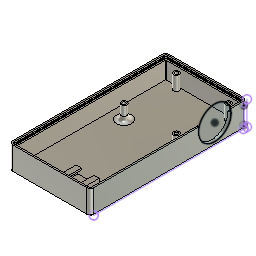
Boitier rover RTK (Autodesk Fusion 360 design; units mm, degrees)
Autodesk Fusion 360 part; units mm, degrees
sketch "Esquisse1" plane through (0, 0, 0) normal (0, 0, 1) x (1, 0, 0) in component "Face Antenne"
  line L0 (32, -67.5) -> (-32, -67.5)
  line L1 (-35, -64.5) -> (-35, 64.5)
  line L2 (-32, 67.5) -> (32, 67.5)
  line L3 (35, 64.5) -> (35, -64.5)
  line L4 (35, -67.5) -> (-35, 67.5) construction
  line L5 (-35, -67.5) -> (35, 67.5) construction
  arc A0 (-32, 67.5) -> (-35, 64.5) centre (-32, 64.5) ccw
  arc A1 (-35, -64.5) -> (-32, -67.5) centre (-32, -64.5) ccw
  arc A2 (32, -67.5) -> (35, -64.5) centre (32, -64.5) ccw
  arc A3 (35, 64.5) -> (32, 67.5) centre (32, 64.5) ccw
  dimension "d31" = 70
  dimension "d32" = 135
  dimension "d33" = 3
  constraint horizontal L0
  constraint perpendicular L0 L1
  constraint parallel L0 L2
  constraint parallel L1 L3
  constraint coincident L4 origin
  constraint coincident L5 origin
  constraint coincident L4.end L2
  constraint coincident L4.end L1
  constraint tangent L2 A0
  constraint tangent L1 A0
  constraint coincident L5.start L1
  constraint coincident L5.start L0
  constraint tangent L1 A1
  constraint tangent L0 A1
  constraint equal A0 A1
  constraint coincident L4.start L3
  constraint coincident L4.start L0
  constraint tangent L3 A2
  constraint tangent L0 A2
  constraint equal A0 A2
  constraint coincident L5.end L3
  constraint coincident L5.end L2
  constraint tangent L3 A3
  constraint tangent L2 A3
  constraint equal A0 A3
  measures "d31" distance of L4.end L5.end
  measures "d32" distance of L5.start L4.end
  measures "d33" radius of A0
extrude "Extrusion1" add sketch "Esquisse1" along normal blind 2.7 makes body 1 in component "Face Antenne"
sketch "Esquisse2" plane through (0, 0, 0) normal (0, 1, 0) x (1, 0, 0) in component "Face Antenne"
  line L0 (35, 0) -> (35, -20.7)
  line L1 (35, -20.7) -> (33.6, -20.7)
  line L2 (33.6, -20.7) -> (33.6, -19.2)
  line L3 (33.6, -19.2) -> (33.8, -19.2)
  line L4 (33.8, -19.2) -> (33.8, -18.2)
  line L5 (33.8, -18.2) -> (33.6, -18.2)
  line L6 (33.6, -18.2) -> (33.6, -17.7)
  line L7 (33.6, -17.7) -> (32.3, -17.7)
  line L8 (32.3, -17.7) -> (32.3, 0)
  line L9 (32.3, 0) -> (35, 0)
  line L10 (35, 0) -> (35, -2.7)
  line L11 (32, 0) -> (-32, 0)
  dimension "d36" = 2.7
  dimension "d37" = 1.4
  dimension "d38" = 1
  dimension "d39" = 0.5
  dimension "d41" = 0.2
  dimension "d42" = 20.7
  dimension "d131" = 1.5
  constraint vertical L0
  constraint perpendicular L0 L1
  constraint perpendicular L1 L2
  constraint perpendicular L2 L3
  constraint perpendicular L3 L4
  constraint perpendicular L4 L5
  constraint perpendicular L5 L6
  constraint perpendicular L6 L7
  constraint perpendicular L7 L8
  constraint perpendicular L0 L9
  constraint collinear L0 L10
  constraint collinear L9 L11
  constraint collinear L2 L6
  measures "d36" distance of L0.start L8.end
  measures "d37" distance of L0.end L1.end
  measures "d38" distance of L3.end L4.end
  measures "d39" distance of L5.end L6.end
  measures "d41" distance of L2.end L3.end
  measures "d42" distance of L0.start L0.end
  measures "d131" distance of L1.end L2.end
sweep "Balayage1" add profiles "Esquisse2" path "Esquisse1" along A2 L0 A1 L1 A0 L2 A3 L3 section 1 bodies 1 in component "Face Antenne"
sketch "Esquisse1 (2)" plane through (0, 0, 0) normal (0, 0, 1) x (1, 0, 0) in component "Face batterie"
  line L0 (-35, -64.5) -> (-35, 64.5)
  line L1 (35, 64.5) -> (35, -64.5)
  line L2 (-32, 67.5) -> (32, 67.5)
  arc A0 (-32, 67.5) -> (-35, 64.5) centre (-32, 64.5) ccw
  arc A1 (35, 64.5) -> (32, 67.5) centre (32, 64.5) ccw
  arc A2 (32, -67.5) -> (35, -64.5) centre (32, -64.5) ccw
  line L3 (32, -67.5) -> (-32, -67.5)
  arc A3 (-35, -64.5) -> (-32, -67.5) centre (-32, -64.5) ccw
  point P0 (-32, 64.5)
extrude "Extrusion1'" add sketch "Esquisse1 (2)" against normal blind 2.7 separate body makes body 2 in component "Face batterie"
sketch "Esquisse2 (2)" plane through (0, 0, 0) normal (0, 1, 0) x (1, 0, 0) in component "Face batterie"
  line L0 (35, 0) -> (35, 19.29)
  line L1 (35, 19.29) -> (33.4, 19.29)
  line L2 (33.4, 22.29) -> (32.3, 22.29)
  line L3 (32.3, 22.29) -> (32.3, 0)
  line L4 (32.3, 0) -> (35, 0)
  line L5 (33.8, 20.8) -> (33.8, 21.8)
  line L6 (32.3, 40) -> (35, 40)
  line L7 (32.3, 22.3) -> (32.3, 40)
  line L8 (32, 0) -> (-32, 0)
  line L9 (33.4, 21.7) -> (33.5, 21.7)
  line L10 (33.7, 21.5) -> (33.7, 21.1)
  line L11 (33.5, 20.9) -> (33.4, 20.9)
  line L12 (33.4, 19.29) -> (33.4, 20.9)
  line L13 (33.4, 21.7) -> (33.4, 22.29)
  line L14 (33.6, 19.3) -> (33.6, 20.8)
  line L15 (35, 19.3) -> (33.6, 19.3)
  line L16 (33.6, 22.3) -> (32.3, 22.3)
  line L17 (33.6, 20.8) -> (33.8, 20.8)
  line L18 (33.8, 21.8) -> (33.6, 21.8)
  arc A0 (33.7, 21.5) -> (33.5, 21.7) centre (33.5, 21.5) ccw
  arc A1 (33.5, 20.9) -> (33.7, 21.1) centre (33.5, 21.1) ccw
  dimension "d151" = 0.01
  dimension "d152" = 0.01
  dimension "d153" = 0.1
  dimension "d154" = 0.1
  dimension "d155" = 0.2
  dimension "d156" = 0.1
  dimension "d157" = 0.2
  constraint vertical L0
  constraint perpendicular L0 L1
  constraint perpendicular L1 L12
  constraint perpendicular L2 L3
  constraint perpendicular L0 L4
  constraint equal L4 L6
  constraint collinear L3 L7
  constraint collinear L4 L8
  constraint coincident L9.start L12
  constraint perpendicular L9 L12
  constraint perpendicular L9 L10
  constraint perpendicular L11 L12
  constraint vertical L13
  constraint coincident L2.end L7
  constraint tangent L9 A0
  constraint tangent L10 A0
  constraint tangent L11 A1
  constraint tangent L10 A1
  constraint equal A0 A1
  measures "d151" distance of L1 L15
  measures "d152" distance of L2 L16
  measures "d153" distance of L11 L17
  measures "d154" distance of L9 L18
  measures "d155" distance of L12 L14
  measures "d156" distance of L5 L10
  measures "d157" radius of A0
sweep "Balayage1'" add profiles "Esquisse2 (2)" path "Esquisse1 (2)" along L1 A1 L2 A0 L0 A3 L3 A2 section 1 bodies 2 in component "Face batterie"
sketch "Esquisse5" plane through (35, 0, 0) normal (1, 0, 0) x (0, 1, 0)
  line L0 (-64.5, 0) -> (64.5, 0)
  line L1 (64.5, 0) -> (64.5, 20.7)
  line L2 (64.5, 20.7) -> (-64.5, 20.7)
  line L3 (-64.5, 20.7) -> (-64.5, 0)
  line L4 (67.5, 0) -> (67.5, 20.7)
  line L5 (64.5, 0) -> (-64.5, 0)
  circle A0 centre (39.8, 17) radius 14
  line L6 (64.8, 2.7) -> (64.8, 17.7)
  line L7 (64.8, 17.7) -> (64.8, 2.7)
  dimension "d222" = 28
  dimension "d223" = 25
  dimension "d224" = 17
  measures "d222" diameter of A0
  measures "d223" distance of A0.centre L6
  measures "d224" distance of L5 A0.centre
extrude "Extrusion7" cut sketch "Esquisse5" against normal up to surface (2.7 mm away) contours L2 A0 | L2 A0 bodies 1 in component "Face Antenne"
extrude "Extrusion4" add sketch "Esquisse1" along normal blind 3 bodies 1 in component "Face Antenne"
sketch "Esquisse6" plane through (0, 0, 3) normal (0, 0, 1) x (-1, 0, 0) in component "Face Antenne"
  arc A0 (-32.3, -64.5) -> (-32, -64.8) centre (-32, -64.5) ccw
  line L0 (-32, -64.8) -> (32, -64.8)
  arc A1 (32, -64.8) -> (32.3, -64.5) centre (32, -64.5) ccw
  line L1 (32.3, -64.5) -> (32.3, 64.5)
  arc A2 (32.3, 64.5) -> (32, 64.8) centre (32, 64.5) ccw
  line L2 (32, 64.8) -> (-32, 64.8)
  arc A3 (-32, 64.8) -> (-32.3, 64.5) centre (-32, 64.5) ccw
  line L3 (-32.3, 64.5) -> (-32.3, -39.8)
  line L4 (-32.3, -39.8) -> (-32.3, -64.5)
  circle A4 centre (20.7, -62.3) radius 2.5
  circle A5 centre (-24.3, -62.3) radius 2.5
  circle A6 centre (20.7, -17.3) radius 2.5
  circle A7 centre (-24.3, -17.3) radius 2.5
  dimension "d87" = 45
  dimension "d88" = 45
  dimension "d90" = 8
  dimension "d211" = 2.5
  constraint equal A4 A5
  constraint equal A4 A6
  constraint equal A6 A7
  constraint vertical A5.centre A7.centre
  constraint vertical A4.centre A6.centre
  constraint horizontal A4.centre A5.centre
  constraint horizontal A6.centre A7.centre
  constraint tangent L0 A5
  measures "d87" distance of A5.centre A7.centre
  measures "d88" distance of A4.centre A5.centre
  measures "d90" distance of L4 A5.centre
  measures "d211" distance of L0 A5.centre
extrude "Extrusion5" add sketch "Esquisse6" along normal blind 12.03 contours A5 | A4 | A6 | A7 bodies 1 in component "Face Antenne"
hole "Perçage1" at (24.3, 62.3, 3) at (-20.7, 62.3, 3) at (24.3, 17.3, 3) at (-20.7, 17.3, 3) direction (0, 0, 1) diameter 2.7 end through all bodies 1 in component "Face Antenne"
fillet "Congé2" radius 4 2 edges at (26.6308, 16.396, 3) (-18.3692, 16.396, 3) on bodies 1 in component "Face Antenne"
sketch "Esquisse7" plane through (0, -64.8, 0) normal (0, 1, 0) x (-1, 0, 0) in component "Face Antenne"
  line L0 (-32, 3) -> (32, 3)
  line L1 (32, 3) -> (32, 17.7)
  line L2 (32, 17.7) -> (-32, 17.7)
  line L3 (-32, 17.7) -> (-32, 3)
  line L4 (-20, 10.3) -> (-15.4, 10.3)
  line L5 (-15.4, 10.3) -> (-15.4, 8.8)
  line L6 (-15.4, 8.8) -> (-18.3, 8)
  line L7 (-18.3, 8) -> (-18.3, 4.5)
  line L8 (-1.7, 4.5) -> (-1.7, 8)
  line L9 (-1.7, 8) -> (-4.6, 8.8)
  line L10 (-4.6, 8.8) -> (-4.6, 10.3)
  line L11 (-4.6, 10.3) -> (0, 10.3)
  line L12 (0, 10.3) -> (0, 3)
  line L13 (0, 3) -> (-20, 3)
  line L14 (-20, 3) -> (-20, 10.3)
  line L15 (-18.3, 4.5) -> (-1.7, 4.5)
  line L16 (-32, 3) -> (32, 3)
  line L17 (-10, 20) -> (-10, -14) construction
  dimension "d98" = 20
  dimension "d100" = 10.8
  dimension "d102" = 16.6
  dimension "d103" = 7.3
  dimension "d105" = 1.5
  dimension "d107" = 1.5
  dimension "d108" = 3.5
  dimension "d132" = 12
  constraint parallel L2 L4
  constraint perpendicular L2 L5
  constraint perpendicular L2 L7
  constraint perpendicular L0 L8
  constraint perpendicular L0 L10
  constraint perpendicular L10 L11
  constraint perpendicular L0 L12
  constraint perpendicular L12 L13
  constraint vertical L14
  constraint equal L12 L14
  constraint equal L4 L11
  constraint equal L5 L10
  constraint equal L7 L8
  constraint collinear L13 L16
  constraint horizontal L15
  constraint vertical L17
  constraint midpoint L13 L17
  constraint symmetric L7.end L8.start L17
  measures "d98" distance of L12.end L13.end
  measures "d100" distance of L5 L10
  measures "d102" distance of L7.end L8.start
  measures "d103" distance of L11.end L12.end
  measures "d105" distance of L13 L15
  measures "d107" distance of L9.end L10.end
  measures "d108" distance of L6.end L7.end
  measures "d132" distance of L3 L14
extrude "Extrusion6" add sketch "Esquisse7" along normal blind 20 contours L0 L4 L5 L6 L7 L8 L9 L10 L11 L12 L13 L14 L15 L16 bodies 1 in component "Face Antenne"
sketch "Esquisse7 (2)" plane through (0, 0, -22.29) normal (0, 0, -1) x (1, 0, 0) in component "Face batterie"
  line L0 (32.3, 64.5) -> (32.3, -64.5)
  line L1 (33.4, -64.5) -> (33.4, 64.5)
  line L2 (35, -64.5) -> (35, 64.5)
  line L3 (33.7, 64.5) -> (33.7, -64.5)
  line L4 (32, 0) -> (-32, 0)
  line L5 (-32, 66.2) -> (-32, 64.8)
  arc A0 (-32, 66.2) -> (-33.7, 64.5) centre (-32, 64.5) ccw
  line L6 (-32.3, 64.5) -> (-33.7, 64.5)
  arc A1 (-32, 64.8) -> (-32.3, 64.5) centre (-32, 64.5) ccw
  arc A2 (-32, 64.8) -> (-32.3, 64.5) centre (-32, 64.5) ccw
  arc A3 (-32, 66.2) -> (-33.7, 64.5) centre (-32, 64.5) ccw
  arc A4 (32, -65.9) -> (33.4, -64.5) centre (32, -64.5) ccw
  arc A5 (32, -66.2) -> (33.7, -64.5) centre (32, -64.5) ccw
  line L7 (32, -66.2) -> (32, -65.9)
  line L8 (33.4, -64.5) -> (33.7, -64.5)
  line L9 (0, -2.5) -> (0, -20)
  line L10 (32, 66.2) -> (32, 64.8)
  arc A6 (33.7, 64.5) -> (32, 66.2) centre (32, 64.5) ccw
  arc A7 (32.3, 64.5) -> (32, 64.8) centre (32, 64.5) ccw
  line L11 (32.3, 64.5) -> (33.7, 64.5)
  arc A8 (32, -66.2) -> (33.7, -64.5) centre (32, -64.5) ccw
  arc A9 (32, -65.9) -> (33.4, -64.5) centre (32, -64.5) ccw
  line L12 (33.4, 64.5) -> (33.4, -64.5)
  arc A10 (-33.7, -64.5) -> (-32, -66.2) centre (-32, -64.5) ccw
  line L13 (-33.4, -64.5) -> (-33.7, -64.5)
  arc A11 (-33.4, -64.5) -> (-32, -65.9) centre (-32, -64.5) ccw
  line L14 (-32, -66.2) -> (-32, -65.9)
  line L15 (0, -2.5) -> (0, -20)
  constraint concentric A0 A1
  constraint concentric A1 A2
  constraint horizontal L6
  constraint coincident A0.end L6.end
  constraint coincident L6.start A1.end
  constraint coincident A0.end A3
  constraint coincident L5.start A0.start
  constraint coincident L5.end A1.start
  constraint vertical L5
  constraint symmetric L5.start L9 L10.start
  constraint symmetric L5.end L9 L10.end
  constraint symmetric A0.end L9 L3.start
  constraint symmetric A0 L9 A6
  constraint symmetric L6.start L9 L0.start
  constraint symmetric A1 L9 A7
  constraint coincident L1.start A4.end
  constraint coincident A5.start L7.start
  constraint coincident A4.start L7.end
  constraint concentric A4 A5
  constraint concentric A5 A8
  constraint coincident L3.end A5.end
  constraint symmetric L1.start L9 L13.start
  constraint symmetric A4.start L9 A11.end
  constraint symmetric A4 L9 A11
  constraint symmetric L3.end L9 A10.start
  constraint symmetric A5.start L9 A10.end
  constraint symmetric A5 L9 A10
  constraint symmetric L15.start L9 L9.start
  constraint symmetric L15.end L9 L9.end
extrude "Extrusion7'" cut sketch "Esquisse7 (2)" against normal up to surface (3 mm away) contours A4 A5 L7 L8 A8 A9 | L10 A6 A7 L11 | L5 A0 L6 A1 A2 A3 | A10 L13 A11 L14 bodies 2 in component "Face batterie"
sketch "Esquisse8" plane through (0, 0, 0) normal (1, 0, 0) x (0, 1, 0) in component "Face batterie"
  line L0 (28.2, -2.7) -> (26.2, -2.7)
  line L1 (26.2, -2.7) -> (26.2, -13.2505)
  line L2 (23.2, -15.7) -> (23.2, -17.7)
  line L3 (23.2, -17.7) -> (26.2, -17.7)
  line L4 (28.2, -15.7) -> (28.2, -2.7)
  arc A0 (23.2, -15.7) -> (26.2, -13.2505) centre (23.7, -13.2505) ccw
  line L5 (64.5, -2.7) -> (-64.5, -2.7)
  arc A1 (26.2, -17.7) -> (28.2, -15.7) centre (26.2, -15.7) ccw
  point P0 (28.2, -17.7)
  point P1 (-64.8, -2.7)
  dimension "d182" = 5
  dimension "d183" = 2
  dimension "d185" = 2
  dimension "d186" = 2.5
  dimension "d187" = 91
  dimension "d188" = 13
  dimension "d210" = 2
  constraint horizontal L0
  constraint perpendicular L0 L1
  constraint perpendicular L2 L3
  constraint vertical L4
  constraint tangent L1 A0
  constraint coincident L2.start A0.start
  constraint horizontal L3
  constraint coincident L0.end L5
  constraint coincident P0 L3
  constraint coincident P0 L4
  constraint tangent L3 A1
  constraint tangent L4 A1
  measures "d182" distance of L2.end P0
  measures "d183" distance of L2.start L2.end
  measures "d185" distance of L0.start L0.end
  measures "d186" radius of A0
  measures "d187" horizontal distance of L0.end P1
  measures "d188" distance of L0 L2.start
  measures "d210" radius of A1
extrude "Extrusion6'" add sketch "Esquisse8" along normal mid plane 10 bodies 2 in component "Face batterie"
fillet "Congé3" radius 2 2 edges at (0, 28.2, -2.7) (0, 26.2, -2.7) on bodies 2 in component "Face batterie"
fillet "Congé4" radius 1 1 faces at (-11.6667, 21.5, 0) on bodies 2 in component "Face batterie"
fillet "Congé3'" radius 1 1 faces at (11.6667, -21.5, 0) on bodies 1 in component "Face Antenne"
extrude "Extrusion9" cut sketch "Esquisse5" against normal blind 2.7 contours L2 A0 | L2 A0 sketch seen with x (1, 0, 0) y (0, 1, 0) z (0, 0, 1) at (0, 0, -40) bodies 2 in component "Face batterie"
component "Face Antenne" placed x (1, 0, 0) y (0, 1, 0) z (0, 0, 1) at (0, 0, 0)
component "Face batterie" placed x (1, 0, 0) y (0, 1, 0) z (0, 0, 1) at (0, 0, 40)
